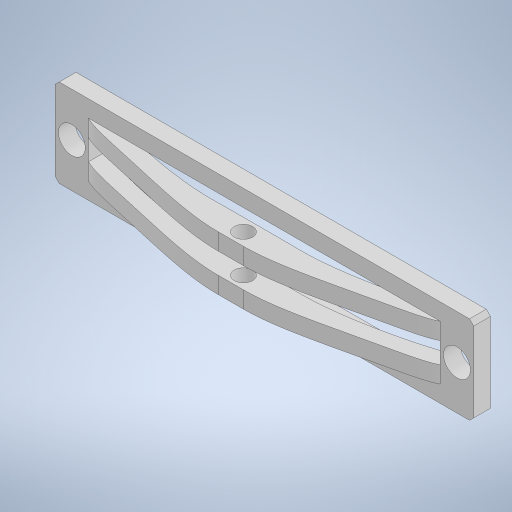
# Autodesk Inventor part: мост
Saved by Autodesk Inventor 2023.1 (Build 271208000, 208)
## iProperties
Created: 2025-12-16
Part Number: мост
Material: Типовые
Document SubType Name: Modeling
Designer: DELL
Density: 1 g/cm^3
Appearance: По умолчанию
Author: DELL
Autodesk Inventor part; units mm, degrees
ref_plane "YZ Plane" through (0, 0, 0) normal (1, 0, 0) x (0, 1, 0)
ref_plane "XZ Plane" through (0, 0, 0) normal (0, 1, 0) x (-1, 0, 0)
ref_plane "XY Plane" through (0, 0, 0) normal (0, 0, 1) x (1, 0, 0)
sketch "Эскиз1" plane through (0, 0, 0) normal (0, 0, 1) x (1, 0, 0)
  line L0 (-30, -12.5) -> (30, -12.5) construction
  line L1 (30, -12.5) -> (30, 12.5) construction
  line L2 (30, 12.5) -> (-30, 12.5) construction
  line L3 (-30, 12.5) -> (-30, -12.5) construction
  line L4 (-30, -12.5) -> (30, 12.5) construction
  line L5 (30, -12.5) -> (-30, 12.5) construction
  line L6 (-25, 5.25) -> (25, 5.25)
  line L7 (25, 5.25) -> (25, -5.25)
  line L8 (25, -5.25) -> (-25, -5.25)
  line L9 (-25, -5.25) -> (-25, 5.25)
  line L10 (-25, 5.25) -> (25, -5.25) construction
  line L11 (25, 5.25) -> (-25, -5.25) construction
  line L12 (21, 3.25) -> (-21, 3.25)
  line L13 (-21, -3.25) -> (21, -3.25)
  line L14 (21, 3.25) -> (21, -3.25)
  line L15 (-21, 3.25) -> (-21, -3.25)
  point P0 (0, 0)
  dimension "d0" = 60
  dimension "d1" = 25
  dimension "d2" = 50
  dimension "d3" = 10.5
  dimension "d4" = 2
  dimension "d15" = 4
  dimension "d16" = 4
  dimension "d27" = 2
  constraints: 32 end point, 5 parallel, 4 midpoint, 4 perpendicular, 2 horizontal
  measures "d0" distance of L2.end L1.end
  measures "d1" distance of L1.end L0.end
  measures "d2" distance of L7.end L8.end
  measures "d3" distance of L6.end L7.end
  measures "d4" distance between parallel lines of L6 L12
  measures "d15" distance between parallel lines of L7 L14
  measures "d16" distance between parallel lines of L9 L15
  measures "d27" distance between parallel lines of L8 L13
extrude "Выдавливание1" add sketch "Эскиз1" along normal blind 2
sketch "Эскиз4" plane through (0, 0, 2) normal (0, 0, 1) x (1, 0, 0)
  circle A0 centre (-23, 0) radius 1.6
  line L0 (-21, -3.25) -> (-21, 3.25) projected
  point P0 (0, 0)
  dimension "d17" = 3.2
  dimension "d18" = 2
  constraints: 1 centre point
  measures "d17" diameter of A0
  measures "d18" distance from line of L0 A0.centre
extrude "Выдавливание3" cut sketch "Эскиз4" against normal blind 3
mirror "Зеркальное отражение2" about plane through (0, 0, 0) normal (1, 0, 0) of "Выдавливание3"
chamfer "Фаска2" distance 0.5 angle 45 4 edges at (25, -5.25, 1) (-25, -5.25, 1) (-25, 5.25, 1) (25, 5.25, 1)
sketch "Эскиз2" plane through (-25, 5.25, 0) normal (0, 1, 0) x (1, 0, 0)
  spline S0 degree 4 poles (46, 0) (42.3251, -1.5041) (33.5066, -3.3836) (31.2881, -3) (28, -3) knots 0 0 0 0 0 1 1 1 1 1
  line L0 (25, 0) -> (25, -3) construction
  line L1 (25, -3) -> (28, -3)
  line L2 (26.5, -6) -> (23.5, -6)
  line L3 (25, -3) -> (25, -6)
  spline S1 degree 4 poles (26.5, -6) (32.4688, -6) (38.7503, -3.3818) (43.4963, -3.2883) (46, -2) knots 0 0 0 0 0 1 1 1 1 1
  circle A0 centre (25, -4.5) radius 1.1
  line L4 (46, 0) -> (46, -2)
  line L5 (50, -2) -> (0, -2) projected
  spline S2 degree 4 poles (4, 0) (7.6749, -1.5041) (16.4934, -3.3836) (18.7119, -3) (22, -3) knots 0 0 0 0 0 1 1 1 1 1
  line L6 (25, -3) -> (22, -3)
  line L7 (23.5, -6) -> (26.5, -6)
  spline S3 degree 4 poles (23.5, -6) (17.5312, -6) (11.2497, -3.3818) (6.5037, -3.2883) (4, -2) knots 0 0 0 0 0 1 1 1 1 1
  line L8 (4, 0) -> (4, -2)
  line L9 (50, 0) -> (0, 0) projected
  point P0 (37.5638, -2.2507)
  point P1 (31.2637, -3)
  point P2 (36.2453, -4.5)
  point P3 (42.8648, -3)
  point P4 (26.5, -3)
  point P5 (38.8382, -2)
  point P6 (12.4362, -2.2507)
  point P7 (18.7363, -3)
  point P8 (13.7547, -4.5)
  point P9 (7.1352, -3)
  point P10 (11.1618, -2)
  point P11 (4, -2)
  point P12 (23.5, -9)
  point P13 (4, -2)
  point P14 (45.3365, 0)
  point P15 (4, 0)
  point P16 (23.5, -3)
  point P17 (26.5, -6)
  dimension "d7" = 3
  dimension "d8" = 2.2
  dimension "d9" = 3
  dimension "d10" = 3
  dimension "d32" = 2
  dimension "d39" = 1
  constraints: 16 end point, 9 symmetric about line, 4 midpoint, 3 perpendicular, 1 centre point, 1 horizontal, 1 point on line, 1 vertical, 17 other
  measures "d7" distance of L0.end L1.end
  measures "d8" diameter of A0
  measures "d9" distance from line of point (26.5, -3) L2
  measures "d10" distance of L2.start L2.end
  measures "d32" distance of L4.start L4.end
  measures "d39" distance from line of L5 point (23.5, -3)
extrude "Выдавливание7" add sketch "Эскиз2" against normal blind 4 contours L4 L5 S0 | L5 S1 L2 L3 A0 L1 S0 | S2 L5 L8 | S2 L6 L3 A0 L2 S3 L5
extrude "Выдавливание8" cut sketch "Эскиз2" against normal blind 2 contours L5 S1 L2 L3 A0 L1 S0 | S2 L6 L3 A0 L2 S3 L5
mirror "Зеркальное отражение5" about plane through (0, 0, 0) normal (0, 1, 0) of "Выдавливание7", "Выдавливание8"
